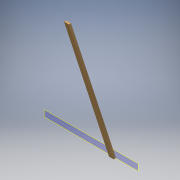
# Autodesk Inventor part: FL-RR Wood Brace
Saved by Autodesk Inventor 2017 (Build 210142000, 142)
## iProperties
Created: 2017-01-22
Part Number: FL-RR Wood Brace
Material: Generic
Document SubType Name: Modeling
Designer: Roksbot
Density: 1 g/cm^3
Appearance: Yellow Pine - Solid Stained Light Low Gloss
Author: Roksbot
Autodesk Inventor part; units mm, degrees
ref_plane "YZ Plane" through (0, 0, 0) normal (1, 0, 0) x (0, 1, 0)
ref_plane "XZ Plane" through (0, 0, 0) normal (0, 1, 0) x (-1, 0, 0)
ref_plane "XY Plane" through (0, 0, 0) normal (0, 0, 1) x (1, 0, 0)
ref_plane "Work Plane1" through (0, 0, -3.175) normal (0, 0, -1) x (-1, 0, 0)
sketch "Sketch1" plane through (0, 0, -3.175) normal (0, 0, -1) x (-1, 0, 0)
  circle A0 centre (171.45, -37.338) radius 2.667 projected
  circle A1 centre (184.15, -11.938) radius 2.667 projected
  circle A2 centre (577.85, 750.062) radius 2.667 construction
  circle A3 centre (565.15, 724.662) radius 2.667 construction
  line L0 (0, 763.524) -> (736.6, 763.524) projected
  line L1 (736.6, -50.8) -> (0, -50.8) projected
  line L2 (154.0806, -50.8) -> (541.7292, 763.524)
  line L3 (582.5194, 763.524) -> (194.8708, -50.8)
  line L4 (194.8708, -50.8) -> (154.0806, -50.8)
  line L5 (541.7292, 763.524) -> (582.5194, 763.524)
  line L6 (487.8257, 564.3774) -> (487.8257, 502.6234) construction
  line L7 (594.2009, 565.5044) -> (496.0553, 565.5044) construction
  line L8 (488.8257, 565.3774) -> (496.0553, 565.3774) construction
  line L9 (248.7743, 148.3466) -> (248.7743, 210.1006) construction
  line L10 (247.7743, 147.3466) -> (240.5447, 147.3466) construction
  line L11 (142.3991, 147.2196) -> (240.5447, 147.2196) construction
  arc A4 (247.7743, 147.3466) -> (248.7743, 148.3466) centre (247.7743, 148.3466) ccw construction
  arc A5 (488.8257, 565.3774) -> (487.8257, 564.3774) centre (488.8257, 564.3774) ccw construction
  line L12 (622.3, 759.587) -> (622.3, 435.737) construction
  line L13 (114.3, -46.863) -> (114.3, 276.987) construction
  circle A6 centre (565.15, 750.062) radius 2.667 projected
  circle A7 centre (552.45, 724.662) radius 2.667 projected
  point P0 (0, 0)
  dimension "d0" = 36.83
  dimension "d1" = 39.7806
  constraints: 16 end point, 6 tangent, 4 horizontal, 4 point on circle, 4 point on line, 2 centre point, 2 parallel, 1 collinear, 8 other
  measures "d0" distance between parallel lines of L3 L2
  measures "d1" distance from line of L13 L2.start
extrude "Extrusion1" add sketch "Sketch1" against normal blind 19.2659
body "Solid1"
